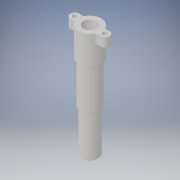
# Autodesk Inventor part: Spacer
Saved by Autodesk Inventor 2019 (Build 230136000, 136)
## iProperties
Created: 2019-10-08
Part Number: Spacer
Material: Generic
Document SubType Name: Modeling
Designer: 19879326
Density: 1 g/cm^3
Appearance: Default
Author: 19879326
Autodesk Inventor part; units mm, degrees
ref_plane "YZ Plane" through (0, 0, 0) normal (1, 0, 0) x (0, 1, 0)
ref_plane "XZ Plane" through (0, 0, 0) normal (0, 1, 0) x (-1, 0, 0)
ref_plane "XY Plane" through (0, 0, 0) normal (0, 0, 1) x (1, 0, 0)
sketch "Sketch1" plane through (0, 0, 0) normal (0, 1, 0) x (-1, 0, 0)
  circle A0 centre (0, 0) radius 4.35
  circle A1 centre (0, 0) radius 7.5
  dimension "d0" = 8.7
  dimension "d4" = 15
  constraints: 2 centre point, 2 coincident
  measures "d0" diameter of A0
  measures "d4" diameter of A1
extrude "Extrusion1" add sketch "Sketch1" along normal blind 75
sketch "Sketch2" plane through (0, 75, 0) normal (0, 1, 0) x (1, 0, 0)
  circle A0 centre (-10, 0) radius 1.5
  circle A1 centre (10, 0) radius 1.5
  circle A2 centre (-10, 0) radius 3
  circle A3 centre (10, 0) radius 3
  point P0 (0, 0)
  dimension "d8" = 3
  dimension "d9" = 20
  dimension "d10" = 10
  dimension "d11" = 6
  constraints: 4 centre point, 2 coincident, 2 equal radius
  measures "d8" diameter of A0
  measures "d9" distance of A1.centre A0.centre
  measures "d10" distance of point (0, 0) A1.centre
  measures "d11" diameter of A2
extrude "Extrusion2" add sketch "Sketch2" against normal blind 6
fillet "Fillet1" radius 2 4 edges at (-7.3625, 72, -1.4295) (-7.3625, 72, 1.4295) (7.3625, 72, -1.4295) (7.3625, 72, 1.4295)
sketch "Sketch3" plane through (0, 0, 0) normal (0, -1, 0) x (1, 0, 0)
  circle A0 centre (0, 0) radius 6.5
  circle A1 centre (0, 0) radius 6.5
  circle A2 centre (0, 0) radius 7.5
  circle A3 centre (0, 0) radius 7.5 projected
  dimension "d15" = 13
  constraints: 3 centre point, 3 coincident, 2 concentric
  measures "d15" diameter of A0
extrude "Extrusion3" cut sketch "Sketch3" against normal blind 55
sketch "Sketch4" plane through (0, 0, 0) normal (0, -1, 0) x (1, 0, 0)
  circle A0 centre (0, 0) radius 5.5
  circle A1 centre (0, 0) radius 6.5
  circle A2 centre (0, 0) radius 6.5 projected
  dimension "d18" = 11
  constraints: 2 centre point, 2 coincident, 1 concentric
  measures "d18" diameter of A0
extrude "Extrusion4" cut sketch "Sketch4" against normal blind 28
chamfer "Chamfer2" distance 1 angle 45 3 edges at (7.5, 55, 0) (-6.5, 28, 0) (-5.5, 0, 0)
body "Solid1"
